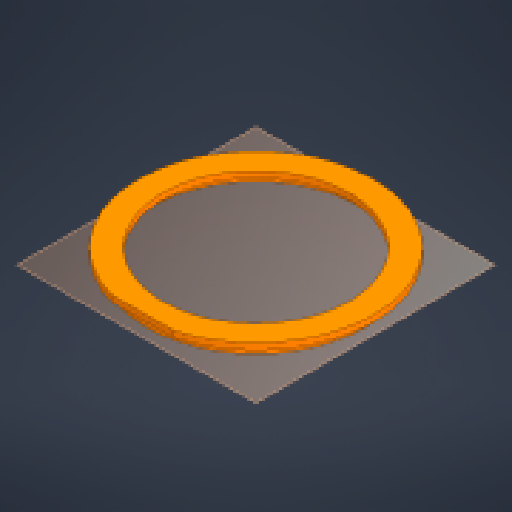
# Autodesk Inventor part: ring
Saved by Autodesk Inventor 2024 (Build 280153000, 153)
## iProperties
Created: 2023-11-07
Part Number: ring
Material: Типовые
Document SubType Name: Modeling
Designer: user
Density: 1 g/cm^3
Appearance: По умолчанию
Author: user
Autodesk Inventor part; units mm, degrees
ref_plane "YZ Plane" through (0, 0, 0) normal (1, 0, 0) x (0, 1, 0)
ref_plane "РабПлоскость1" through (0, 0, -3) normal (0, 0, 1) x (1, 0, 0)
sketch "Эскиз1" plane through (0, 0, -3) normal (0, 0, 1) x (1, 0, 0)
  circle A0 centre (0, 0) radius 33.125 projected
  arc A1 (-2.5, 35.0359) -> (2.5, 35.0359) centre (0, 0) ccw projected
  line L0 (2.5, 37.9177) -> (2.5, 35.0359)
  line L1 (-2.5, 35.0359) -> (-2.5, 37.9177)
  arc A2 (2.5, 37.9177) -> (-2.5, 37.9177) centre (0, 0) ccw
  point P0 (2.5, 35.0359)
  constraints: 4 end point, 3 point on circle, 2 vertical, 1 centre point, 6 other
ref_plane "РабПлоскость2" through (-38, -36.68, 0) normal (0, 0, 1) x (1, 0, 0)
extrude "Выдавливание1" add sketch "Эскиз1" along normal up to surface (3 mm away)
sketch "Эскиз2" plane through (0, 0, 0) normal (0, 0, 1) x (1, 0, 0)
  circle A0 centre (0, 0) radius 30.25 projected
  arc A1 (-2.5, 37.9177) -> (-9.9286, -36.68) centre (0, 0) ccw projected
  arc A2 (9.9286, -36.68) -> (2.5, 37.9177) centre (0, 0) ccw projected
  arc A3 (2.5, 37.9177) -> (-2.5, 37.9177) centre (0, 0) ccw
  line L0 (9.9286, -36.68) -> (-9.9286, -36.68)
  point P0 (-2.5, 37.9177)
  constraints: 3 point on circle, 2 end point, 1 centre point, 1 concentric, 1 horizontal
extrude "Выдавливание2" add sketch "Эскиз2" along normal blind 2
